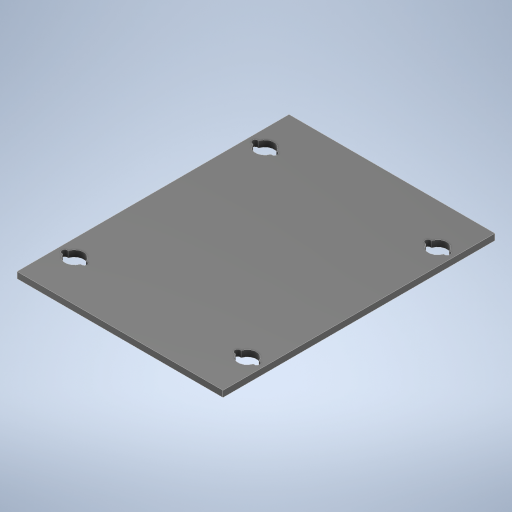
# Autodesk Inventor part: SUSTAINA-AUDIO-BOARD
Saved by Autodesk Inventor 2024.2 (Build 282272000, 272)
## iProperties
Created: 2024-06-01
Part Number: SUSTAINA-AUDIO-BOARD
Material: Generic
Document SubType Name: Modeling
Designer: Masato Kubotera
Density: 1 g/cm^3
Appearance: Smooth - Black
Author: Masato Kubotera
Autodesk Inventor part; units mm, degrees
ref_plane "YZ Plane" through (0, 0, 0) normal (1, 0, 0) x (0, 1, 0)
ref_plane "XZ Plane" through (0, 0, 0) normal (0, 1, 0) x (-1, 0, 0)
ref_plane "XY Plane" through (0, 0, 0) normal (0, 0, 1) x (1, 0, 0)
sketch "Sketch1" plane through (0, 0, 0) normal (0, 0, 1) x (1, 0, 0)
  line L0 (-35, -26.5) -> (35, -26.5)
  line L1 (35, -26.5) -> (35, 26.5)
  line L2 (35, 26.5) -> (-35, 26.5)
  line L3 (-35, 26.5) -> (-35, -26.5)
  line L4 (-35, -26.5) -> (35, 26.5) construction
  line L5 (35, -26.5) -> (-35, 26.5) construction
  line L6 (-24.5, -22.25) -> (24.5, -22.25) construction
  line L7 (24.5, -22.25) -> (24.5, 22.25) construction
  line L8 (24.5, 22.25) -> (-24.5, 22.25) construction
  line L9 (-24.5, 22.25) -> (-24.5, -22.25) construction
  line L10 (-24.5, -22.25) -> (24.5, 22.25) construction
  line L11 (24.5, -22.25) -> (-24.5, 22.25) construction
  circle A0 centre (24.5, -22.25) radius 2.4
  arc A1 (23.7801, -24.5395) -> (25.2199, -24.5395) centre (24.5, -24.75) ccw
  arc A2 (25.2199, -19.9605) -> (23.7801, -19.9605) centre (24.5, -19.75) ccw
  line L12 (0, -26.5) -> (0, 26.5) construction
  line L13 (-35, 0) -> (35, 0) construction
  circle A3 centre (-24.5, -22.25) radius 2.4
  arc A4 (-25.2199, -24.5395) -> (-23.7801, -24.5395) centre (-24.5, -24.75) ccw
  arc A5 (-23.7801, -19.9605) -> (-25.2199, -19.9605) centre (-24.5, -19.75) ccw
  circle A6 centre (24.5, 22.25) radius 2.4
  arc A7 (25.2199, 24.5395) -> (23.7801, 24.5395) centre (24.5, 24.75) ccw
  arc A8 (23.7801, 19.9605) -> (25.2199, 19.9605) centre (24.5, 19.75) ccw
  arc A9 (-23.7801, 24.5395) -> (-25.2199, 24.5395) centre (-24.5, 24.75) ccw
  circle A10 centre (-24.5, 22.25) radius 2.4
  arc A11 (-25.2199, 19.9605) -> (-23.7801, 19.9605) centre (-24.5, 19.75) ccw
  point P0 (0, 0)
  point P1 (24.5, -19)
  point P2 (24.5, -25.5)
  point P3 (25.2199, 19.9605)
  point P4 (23.7801, 19.9605)
  point P5 (-25.2199, -19.9605)
  point P6 (-23.7801, -19.9605)
  point P7 (23.7801, -19.9605)
  point P8 (25.2199, -19.9605)
  point P9 (-23.7801, 19.9605)
  point P10 (-25.2199, 19.9605)
  dimension "d32" = 70
  dimension "d33" = 53
  dimension "d34" = 4.8
  dimension "d35" = 6.5
  dimension "d36" = 1.5
  dimension "d38" = 8.5
  dimension "d41" = 49
  constraints: 28 end point, 26 point on circle, 24 symmetric about line, 12 centre point, 8 midpoint, 4 parallel, 2 horizontal, 2 perpendicular, 1 coincident, 1 point on line, 10 other
  measures "d32" distance of L2.end L1.end
  measures "d33" distance of L1.end L0.end
  measures "d34" diameter of A0
  measures "d35" distance of point (24.5, -19) point (24.5, -25.5)
  measures "d36" diameter of A1
  measures "d38" diameter of L0 L6
  measures "d41" distance of L6.start L6.end
extrude "Extrusion1" add sketch "Sketch1" along normal blind 1.6
body "Solid3"
